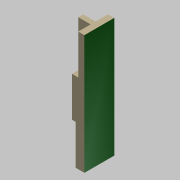
# Autodesk Inventor part: Hill
Saved by Autodesk Inventor 2015 (Build 190159000, 159)
## iProperties
Created: 2015-03-07
Part Number: Hill
Material: Generic
Document SubType Name: Modeling
Designer: Vukica
Density: 1 g/cm^3
Appearance: Plywood - Weathered
Author: Vukica
Autodesk Inventor part; units mm, degrees
ref_plane "YZ Plane" through (0, 0, 0) normal (1, 0, 0) x (0, 1, 0)
ref_plane "XZ Plane" through (0, 0, 0) normal (0, 1, 0) x (-1, 0, 0)
ref_plane "XY Plane" through (0, 0, 0) normal (0, 0, 1) x (1, 0, 0)
sketch "Sketch1" plane through (0, 0, 0) normal (0, 0, 1) x (1, 0, 0)
  line L0 (0, 0) -> (127, 0)
  line L1 (127, 0) -> (127, 2438.4)
  line L2 (127, 2438.4) -> (0, 2438.4)
  line L3 (0, 2438.4) -> (0, 0)
  dimension "d0" = 127
  dimension "d1" = 2438.4
  constraints: 8 end point, 2 parallel, 1 horizontal, 1 perpendicular
  measures "d0" distance of L1.end L2.end
  measures "d1" distance of L0.end L1.end
extrude "Extrusion1" add sketch "Sketch1" along normal blind 609.6
sketch "Sketch3" plane through (0, 0, 0) normal (-1, 0, 0) x (0, 0, 1)
  line L0 (609.6, 2438.4) -> (609.6, 0) projected
  line L1 (0, 2438.4) -> (0, 0) projected
  line L2 (0, 0) -> (609.6, 0) projected
  line L3 (609.6, 0) -> (609.6, 2438.4) projected
  line L4 (0, 0) -> (609.6, 0)
  line L5 (609.6, 0) -> (609.6, 812.8)
  line L6 (609.6, 812.8) -> (0, 812.8)
  line L7 (0, 812.8) -> (0, 0)
  dimension "d8" = 812.8
  constraints: 8 end point, 2 parallel, 1 horizontal, 1 perpendicular, 1 point on line
  measures "d8" distance between parallel lines of L2 L6
extrude "Extrusion3" add sketch "Sketch3" along normal blind 50.8
sketch "Sketch4" plane through (0, 2438.4, 0) normal (-1, 0, 0) x (0, 0, 1)
  line L0 (609.6, -1625.6) -> (0, -1625.6) projected
  line L1 (609.6, 0) -> (609.6, -1625.6) projected
  line L2 (0, 0) -> (0, -1625.6) projected
  line L3 (0, -1625.6) -> (609.6, -1625.6)
  line L4 (609.6, -1625.6) -> (609.6, -812.8)
  line L5 (609.6, -812.8) -> (0, -812.8)
  line L6 (0, -812.8) -> (0, -1625.6)
  point P0 (0, -2438.4)
  dimension "d11" = 812.8
  constraints: 8 end point, 2 parallel, 1 horizontal, 1 midpoint, 1 perpendicular
  measures "d11" distance between parallel lines of L5 L0
extrude "Extrusion4" add sketch "Sketch4" along normal blind 127
sketch "Sketch5" plane through (0, 1625.6, 0) normal (-1, 0, 0) x (0, 0, 1)
  line L0 (519.5823, 575.5562) -> (519.5823, 226.8611) construction
  line L1 (519.5823, 226.8611) -> (23.9628, 226.8611) construction
  line L2 (23.9628, 226.8611) -> (23.9628, 575.5562) construction
  line L3 (23.9628, 575.5562) -> (519.5823, 575.5562) construction
  point P0 (0, -1625.6)
  constraints: 2 other
sketch "Sketch6" plane through (-127, 2438.4, 0) normal (-1, 0, 0) x (0, 0, 1)
  line L0 (504.953, -1049.3947) -> (504.953, -1386.624) construction
  line L1 (504.953, -1386.624) -> (88.8121, -1386.624) construction
  line L2 (88.8121, -1386.624) -> (88.8121, -1049.3947) construction
  line L3 (88.8121, -1049.3947) -> (504.953, -1049.3947) construction
  point P0 (0, -2438.4)
  constraints: 2 other
sketch "Sketch7" plane through (-50.8, 0, 0) normal (-1, 0, 0) x (0, 0, 1)
  line L0 (510.0659, 619.5124) -> (510.0659, 275.8757) construction
  line L1 (510.0659, 275.8757) -> (79.0869, 275.8757) construction
  line L2 (79.0869, 275.8757) -> (79.0869, 619.5124) construction
  line L3 (79.0869, 619.5124) -> (510.0659, 619.5124) construction
  point P0 (0, 0)
  constraints: 2 other
sketch "Sketch8" plane through (-50.8, 0, 0) normal (-1, 0, 0) x (0, 0, 1)
  line L0 (0, 812.8) -> (609.6, 812.8) projected
  line L1 (0, 0) -> (609.6, 0) projected
  line L2 (355.6, 812.8) -> (254, 812.8)
  line L3 (254, 812.8) -> (254, 0)
  line L4 (254, 0) -> (355.6, 0)
  line L5 (355.6, 0) -> (355.6, 812.8)
  line L6 (609.6, 0) -> (609.6, 812.8) projected
  line L7 (0, 812.8) -> (0, 0) projected
  point P0 (127, 0)
  point P1 (482.6, 0)
  point P2 (609.6, 127)
  point P3 (0, 127)
  dimension "d15" = 254
  dimension "d16" = 254
  constraints: 8 end point, 2 parallel, 2 point on line, 1 horizontal, 1 perpendicular
  measures "d15" distance between parallel lines of L5 L6
  measures "d16" distance between parallel lines of L7 L3
extrude "Extrusion5" add sketch "Sketch8" along normal up to surface (76.2 mm away) contours L0 L5 L1 L3
sketch "Sketch9" plane through (-127, 2438.4, 0) normal (-1, 0, 0) x (0, 0, 1)
  line L0 (254, -2438.4) -> (254, -1625.6) projected
  line L1 (355.6, -1625.6) -> (355.6, -2438.4) projected
  line L2 (609.6, -812.8) -> (0, -812.8) projected
  line L3 (355.6, -1625.6) -> (254, -1625.6)
  line L4 (254, -1625.6) -> (254, -812.8)
  line L5 (254, -812.8) -> (355.6, -812.8)
  line L6 (355.6, -812.8) -> (355.6, -1625.6)
  point P0 (0, -2438.4)
  constraints: 8 end point, 2 parallel, 2 point on line, 1 horizontal, 1 perpendicular
extrude "Extrusion6" add sketch "Sketch9" along normal blind 127
sketch "Sketch10" plane through (0, 1625.6, 0) normal (-1, 0, 0) x (0, 0, 1)
  line L0 (254, 0) -> (254, -812.8) projected
  line L1 (355.6, -812.8) -> (355.6, 0) projected
  line L2 (355.6, 0) -> (254, 0) projected
  line L3 (0, 812.8) -> (609.6, 812.8) projected
  line L4 (355.6, 0) -> (254, 0)
  line L5 (254, 0) -> (254, 812.8)
  line L6 (254, 812.8) -> (355.6, 812.8)
  line L7 (355.6, 812.8) -> (355.6, 0)
  point P0 (0, -1625.6)
  point P1 (127, 812.8)
  point P2 (482.6, 812.8)
  constraints: 8 end point, 2 parallel, 2 point on line, 1 horizontal, 1 perpendicular
extrude "Extrusion7" add sketch "Sketch10" along normal up to surface (254 mm away)
sketch "Sketch11" plane through (-127, 2438.4, 0) normal (-1, 0, 0) x (0, 0, 1)
  line L0 (254, -1625.6) -> (355.6, -1625.6) projected
  line L1 (254, -2438.4) -> (254, -1625.6) projected
  line L2 (355.6, -1625.6) -> (355.6, -2438.4) projected
  line L3 (355.6, -2438.4) -> (254, -2438.4) projected
  point P0 (0, -2438.4)
extrude "Extrusion8" add sketch "Sketch11" along normal up to surface (127 mm away)
sketch "Sketch12" plane through (-50.8, 0, 355.6) normal (0, 0, 1) x (1, 0, 0)
  circle A0 centre (-177.8, 25.4) radius 2.54
  line L0 (0, 0) -> (-203.2, 0) projected
  line L1 (-203.2, 2438.4) -> (-203.2, 0) projected
  circle A1 centre (-152.4, 25.4) radius 2.54
  circle A2 centre (-127, 25.4) radius 2.54
  circle A3 centre (-101.6, 25.4) radius 2.54
  circle A4 centre (-76.2, 25.4) radius 2.54
  circle A5 centre (-50.8, 25.4) radius 2.54
  point P0 (50.8, 0)
  dimension "d25" = 25.4
  dimension "d26" = 25.4
  dimension "d27" = 5.08
  dimension "d30" = 25.4
  constraints: 6 centre point, 1 horizontal, 10 other
  measures "d25" distance from line of L0 A0.centre
  measures "d26" distance from line of L1 A0.centre
  measures "d27" diameter of A0
  measures "d30" distance of A0.centre A1.centre
ref_plane "Work Plane1" through (-50.8, 1219.2, 482.6) normal (0, -1, 0) x (1, 0, 0)
ref_plane "Work Plane2" through (0, 0, 304.8) normal (0, 0, 1) x (1, 0, 0)
mirror "Mirror2" about plane through (0, 0, 304.8) normal (0, 0, 1) of "Extrusion8"
extrude "Extrusion10" cut sketch "Sketch12" against normal blind 12.7
mirror "Mirror3" about plane through (0, 0, 304.8) normal (0, 0, 1) of "Extrusion10"
sketch "Sketch14" plane through (-50.8, 0, 355.6) normal (0, 0, 1) x (1, 0, 0)
  circle A0 centre (-177.8, 2413) radius 2.54
  line L0 (50.8, 2438.4) -> (-203.2, 2438.4) projected
  line L1 (-203.2, 2438.4) -> (-203.2, 0) projected
  circle A1 centre (-152.4, 2413) radius 2.54
  circle A2 centre (-127, 2413) radius 2.54
  circle A3 centre (-101.6, 2413) radius 2.54
  circle A4 centre (-76.2, 2413) radius 2.54
  circle A5 centre (-50.8, 2413) radius 2.54
  point P0 (50.8, 0)
  dimension "d43" = 25.4
  dimension "d44" = 25.4
  dimension "d45" = 5.08
  dimension "d48" = 25.4
  constraints: 6 centre point, 1 horizontal, 10 other
  measures "d43" distance from line of L0 A0.centre
  measures "d44" distance from line of L1 A0.centre
  measures "d45" diameter of A0
  measures "d48" distance of A0.centre A1.centre
extrude "Extrusion11" cut sketch "Sketch14" against normal blind 12.7
mirror "Mirror4" about plane through (0, 0, 304.8) normal (0, 0, 1) of "Extrusion11"
equation "\"d8\" = 0.333333 * d1"
equation "\"d11\" = 0.333333 * d1"
body "Solid1"
